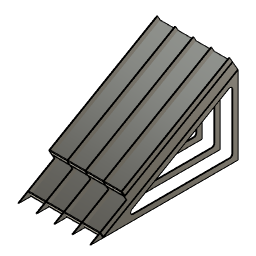
Parts_holder v9 (Autodesk Fusion 360 design; units mm, degrees)
Autodesk Fusion 360 part; units mm, degrees
note: some values were not read from the file. Set by a fixed rule: which sketch regions a step uses.
sketch "Sketch1" plane through (0, 0, 0) normal (0, 0, 1) x (1, 0, 0)
  line L0 (0, 0) -> (270, 0)
  line L1 (270, 0) -> (270, 463)
  line L2 (270, 463) -> (0, 463)
  line L3 (0, 463) -> (0, 0)
  line L4 (600.1429, 643.7143) -> (330.1429, 643.7143)
  line L5 (330.1429, 643.7143) -> (330.1429, 65.7143)
  line L6 (330.1429, 65.7143) -> (600.1429, 65.7143)
  line L7 (600.1429, 65.7143) -> (600.1429, 643.7143)
  line L8 (956.8565, -10.3094) -> (1090.9494, 67.1092)
  line L9 (956.8565, -10.3094) -> (1115, -10.3094) construction
  line L10 (1090.9494, 67.1092) -> (1070.9494, 101.7502)
  line L11 (1070.9494, 101.7502) -> (1471.9192, 333.2502)
  line L12 (991.3565, 9.6092) -> (1002.8565, -10.3094)
  line L13 (991.3565, 9.6092) -> (957.8576, 9.6092) construction
  line L14 (1002.8565, -10.3094) -> (1503.4192, 278.6906)
  line L15 (1002.8565, -10.3094) -> (1306.0004, -10.3094) construction
  line L16 (1503.4192, 278.6906) -> (1520, 278.6906) construction
  line L17 (1503.4192, 278.6906) -> (1503.4192, -10.3094)
  line L18 (956.8565, -10.3094) -> (1503.4192, -10.3094)
  line L19 (1114.818, 9.6906) -> (1473.4192, 9.6906)
  line L20 (1483.4192, 226.7291) -> (1483.4192, 19.6906)
  line L21 (1109.818, 28.3508) -> (1468.4192, 235.3893)
  arc A0 (1109.818, 28.3508) -> (1114.818, 9.6906) centre (1114.818, 19.6906) ccw
  arc A1 (1483.4192, 226.7291) -> (1468.4192, 235.3893) centre (1473.4192, 226.7291) ccw
  arc A2 (1473.4192, 9.6906) -> (1483.4192, 19.6906) centre (1473.4192, 19.6906) ccw
  line L22 (1471.9192, 333.2502) -> (1503.4192, 278.6906)
  line L23 (270, 463) -> (267, 463)
  line L24 (267, 463) -> (267, 405.125)
  line L25 (267, 405.125) -> (270, 405.125)
  line L26 (270, 405.125) -> (270, 463)
  line L27 (270, 347.25) -> (267, 347.25)
  line L28 (267, 347.25) -> (267, 405.125)
  line L29 (267, 289.375) -> (270, 289.375)
  line L30 (267, 347.25) -> (267, 289.375)
  line L31 (270, 231.5) -> (267, 231.5)
  line L32 (267, 231.5) -> (267, 289.375)
  line L33 (267, 173.625) -> (270, 173.625)
  line L34 (267, 231.5) -> (267, 173.625)
  line L35 (270, 115.75) -> (267, 115.75)
  line L36 (267, 115.75) -> (267, 173.625)
  line L37 (267, 57.875) -> (270, 57.875)
  line L38 (267, 115.75) -> (267, 57.875)
  line L39 (270, 0) -> (267, 0)
  line L40 (267, 0) -> (267, 57.875)
  line L41 (267, 463) -> (235.125, 463)
  line L42 (235.125, 463) -> (235.125, 455)
  line L43 (200.25, 115.75) -> (203.25, 115.75)
  line L44 (200.25, 405.125) -> (200.25, 463)
  line L45 (200.25, 463) -> (203.25, 463)
  line L46 (203.25, 463) -> (203.25, 405.125)
  line L47 (203.25, 347.25) -> (203.25, 289.375)
  line L48 (200.25, 347.25) -> (203.25, 347.25)
  line L49 (203.25, 347.25) -> (203.25, 405.125)
  line L50 (203.25, 289.375) -> (200.25, 289.375)
  line L51 (203.25, 231.5) -> (203.25, 289.375)
  line L52 (203.25, 405.125) -> (200.25, 405.125)
  line L53 (200.25, 0) -> (200.25, 463)
  line L54 (203.25, 463) -> (235.125, 463)
  line L55 (203.25, 115.75) -> (203.25, 173.625)
  line L56 (200.25, 231.5) -> (203.25, 231.5)
  line L57 (203.25, 115.75) -> (203.25, 57.875)
  line L58 (203.25, 0) -> (203.25, 57.875)
  line L59 (200.25, 0) -> (203.25, 0)
  line L60 (203.25, 231.5) -> (203.25, 173.625)
  line L61 (203.25, 57.875) -> (200.25, 57.875)
  line L62 (203.25, 173.625) -> (200.25, 173.625)
  point P0 (330.1429, 65.7143)
  dimension "d1" = 270
  dimension "d2" = 463
  dimension "d3" = 270
  dimension "d4" = 578
  dimension "d6" = 30
  dimension "d7" = 40
  dimension "d8" = 463
  dimension "d18" = 60
  dimension "d19" = 23
  dimension "d20" = 30
  dimension "d21" = 578
  dimension "d39" = 10
  dimension "d40" = 10
  dimension "d41" = 10
  dimension "d42" = 115
  dimension "d43" = 3
  dimension "d44" = 57.875
  dimension "d45" = 31.875
  constraint horizontal L0
  constraint vertical L1
  constraint horizontal L2
  constraint vertical L3
  constraint coincident L0.start L3.end
  constraint horizontal L6
  constraint vertical L7
  constraint horizontal L4
  constraint vertical L5
  constraint coincident P0 L5.end
  constraint horizontal L9
  constraint perpendicular L8 L10
  constraint perpendicular L10 L11
  constraint horizontal L13
  constraint coincident L8 L12.start
  constraint coincident L9 L12.end
  constraint horizontal L15
  constraint horizontal L16
  constraint vertical L17
  constraint perpendicular L17 L18
  constraint tangent L21 A0
  constraint tangent L19 A0
  constraint tangent L21 A1
  constraint tangent L20 A1
  constraint tangent L20 A2
  constraint tangent L19 A2
  constraint horizontal L23
  constraint vertical L24
  constraint horizontal L25
  constraint vertical L26
  constraint symmetric L1.end L25 L27.start
  constraint symmetric L23.end L25 L27.end
  constraint symmetric L24.end L25 L28.end
  constraint symmetric L24.end L27 L29.start
  constraint symmetric L25.end L27 L29.end
  constraint symmetric L28.start L27 L30.start
  constraint symmetric L27 L24.end L29.start
  constraint symmetric L27.start L29 L31.start
  constraint symmetric L27.end L29 L31.end
  constraint symmetric L29 L27.end L31.end
  constraint symmetric L29 L30.end L32.end
  constraint symmetric L29.start L31 L33.start
  constraint symmetric L29.end L31 L33.end
  constraint symmetric L31 L32.start L34.start
  constraint symmetric L31 L29.start L33.start
  constraint symmetric L31.start L33 L35.start
  constraint symmetric L31.end L33 L35.end
  constraint symmetric L33 L31.end L35.end
  constraint symmetric L33 L34.end L36.end
  constraint symmetric L33.start L35 L37.start
  constraint symmetric L33.end L35 L37.end
  constraint symmetric L35 L36.start L38.start
  constraint symmetric L35 L33.start L37.start
  constraint symmetric L35.start L37 L0.end
  constraint symmetric L35.end L37 L39.end
  constraint symmetric L37 L35.end L39.end
  constraint symmetric L37 L38.end L40.end
  constraint perpendicular L24 L41
  constraint perpendicular L41 L42
  constraint symmetric L0.end L42 L53.start
  constraint symmetric L1.end L42 L44.end
  constraint symmetric L23.end L42 L45.end
  constraint symmetric L24.end L42 L46.end
  constraint symmetric L25.end L42 L44.start
  constraint symmetric L27.start L42 L48.start
  constraint symmetric L27.end L42 L47.start
  constraint symmetric L29.start L42 L47.end
  constraint symmetric L29.end L42 L50.end
  constraint symmetric L31.start L42 L56.start
  constraint symmetric L31.end L42 L51.start
  constraint symmetric L33.start L42 L55.end
  constraint symmetric L33.end L42 L62.end
  constraint symmetric L35.start L42 L43.start
  constraint symmetric L35.end L42 L43.end
  constraint symmetric L37.start L42 L57.end
  constraint symmetric L37.end L42 L61.end
  constraint symmetric L39.end L42 L58.start
  constraint symmetric L41.end L42 L54.end
  measures "d1" distance of L0.start L0.end
  measures "d2" distance of L0.start L2.end
  measures "d3" distance of P0 L6.end
  measures "d4" distance of P0 L4.end
  measures "d6" angle of L8 L9
  measures "d7" distance of L8.end L10.end
  measures "d8" distance of L10.end L11.end
  measures "d18" angle of L12 L13
  measures "d19" distance of L12.start L12.end
  measures "d20" angle of L14 L15
  measures "d21" distance of L12.end L14.end
  measures "d39" radius of A0
  measures "d40" radius of A1
  measures "d41" radius of A2
  measures "d42" distance of L10 L12
  measures "d43" distance of L1.end L23.end
  measures "d44" distance of L23.end L24.end
  measures "d45" distance of L23.end L41.end
extrude "Extrude2" add sketch "Sketch1" along normal blind 3 makes body 1 at (90, 154.3333, 0) makes body 2 at (420.1429, 258.381, 0) makes body 3 at (1337.0959, 223.4632, 0)
move_body "Move7" bodies 1 2 to x (1, 0, 0) y (0, 0.866025, 0.5) z (0, -0.5, 0.866025) at (0, 32.5151, -115.3481)
move_body "Move8" bodies 3 to x (0, 1, 0) y (0, 0, 1) z (1, 0, 0) at (1428.1435, -1217.8595, -210.284)
move_body "Align4" bodies 3 to x (1, 0, 0) y (0, 1, 0) z (0, 0, 1) at (-828.0006, 350.4284, 138.1025)
move_body "Move9" bodies 3 to x (1, 0, 0) y (0, 1, 0) z (0, 0, 1) at (0, -46, 0)
move_body "Align5" bodies 1 to x (1, 0, 0) y (0, 1, 0) z (0, 0, 1) at (330.1429, 126.5032, 142.3187)
move_body "Move11" bodies 3 to x (1, 0, 0) y (0, 1, 0) z (0, 0, 1) at (-3, 0, 0)
move_body "Move12" bodies 1 to x (1, 0, 0) y (0, 1, 0) z (0, 0, 1) at (0, 10, -17.3205)
pattern_path "PathPattern3" count 5 spacing 66.7496 from (598.6912, 87.9254, -79.8929) along 1 edges at (465.1429, 87.9254, -79.8929) of bodies 3 on bodies 2 makes body 4 at (530.3933, 423.6648, 151.2817) makes body 5 at (463.6437, 423.6648, 151.2817) makes body 6 at (396.8941, 423.6648, 151.2817) makes body 7 at (330.1445, 423.6648, 151.2817)
sketch "Sketch2" plane through (0, 56.576, -97.9924) normal (0, -0.5, 0.866025) x (1, 0, 0)
  line L0 (330.1429, 614.1992) -> (330.1429, 151.1992)
  line L1 (330.1429, 151.1992) -> (600.1429, 151.1992)
  line L2 (600.1429, 151.1992) -> (600.1429, 614.1992)
  line L3 (600.1429, 614.1992) -> (330.1429, 614.1992)
  line L4 (330.1429, 151.1992) -> (330.1429, 154.1992)
  line L5 (330.1429, 151.1992) -> (600.1429, 151.1992)
  line L6 (600.1429, 151.1992) -> (600.1429, 154.1992)
  line L7 (600.1429, 154.1992) -> (330.1429, 154.1992)
  dimension "d31" = 3
  dimension "d32" = 3
  constraint coincident L0.end L1.start
  constraint perpendicular L1 L4
  constraint coincident L1.end L2.start
  constraint perpendicular L1 L6
  measures "d31" distance of L0.end L4.end
  measures "d32" distance of L1.end L6.end
extrude "Extrude3" add sketch "Sketch2" along normal blind 20 separate body contours L0 L1 L2 L4 L5 L6 L7 makes body 8
sketch "Sketch3" plane through (0, 58.076, -100.5905) normal (0, 0.5, -0.866025) x (-1, 0, 0)
  line L0 (-600.1429, 614.1992) -> (-600.1429, 36.1992)
  line L1 (-600.1429, 36.1992) -> (-330.1429, 36.1992)
  line L2 (-330.1429, 36.1992) -> (-330.1429, 614.1992)
  line L3 (-330.1429, 614.1992) -> (-600.1429, 614.1992)
  line L4 (-330.1429, 36.1992) -> (-600.1429, 36.1992)
  line L5 (-600.1429, 36.1992) -> (-600.1429, 39.1992)
  line L6 (-600.1429, 39.1992) -> (-330.1429, 39.1992)
  line L7 (-330.1429, 39.1992) -> (-330.1429, 36.1992)
  dimension "d35" = 3
  constraint coincident L1.end L2.start
  constraint coincident L0.end L1.start
  constraint perpendicular L4 L5
  constraint coincident L2 L6.end
  constraint perpendicular L2 L6
  measures "d35" distance of L0.end L5.end
extrude "Extrude4" add sketch "Sketch3" against normal blind 23 separate body contours L0 L1 L2 L4 L5 L6 L7 makes body 9
move_body "Move13" bodies 8 to x (1, 0, 0) y (0, 1, 0) z (0, 0, 1) at (0, -20, 34.641)
equation "d1 = d3"
equation "d2 = ( 115 * 4 ) * 1 mm + 3 mm"
equation "d3 = ( 60 * 4 ) * 1 mm + ( 3 * 5 ) * 1 mm + ( 3 * 5 ) * 1 mm"
equation "d4 = ( 115 * 5 ) * 1 mm + 3 mm"
equation "d7 = 60 mm - d19 + Mat_thicc"
equation "d8 = d2"
equation "d19 = 20 mm + Mat_thicc"
equation "d21 = d4"
equation "Mat_thicc = 3 mm"
equation "d25 = Mat_thicc"
equation "d44 = d2 / 8"
equation "d45 = ( 63.75 / 2 ) * 1 mm"
